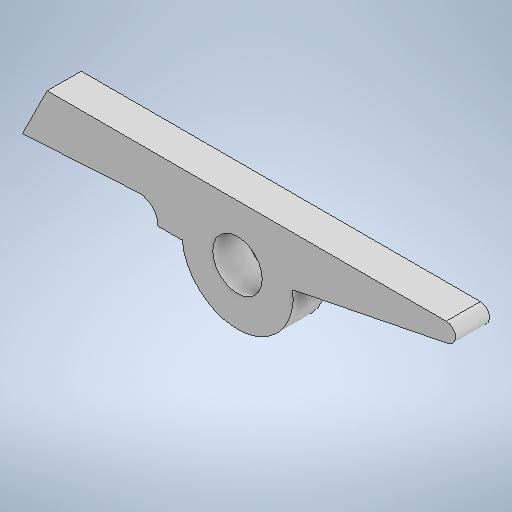
# Autodesk Inventor part: Pieza 4
Saved by Autodesk Inventor 2025.3 (Build 293356030, 356C)
## iProperties
Created: 2025-08-24
Part Number: Pieza 4
Material: Generic
Document SubType Name: Modeling
Designer: PC
Density: 1 g/cm^3
Appearance: Default
Author: PC
Autodesk Inventor part; units mm, degrees
ref_plane "YZ Plane" through (0, 0, 0) normal (1, 0, 0) x (0, 1, 0)
ref_plane "XZ Plane" through (0, 0, 0) normal (0, 1, 0) x (-1, 0, 0)
ref_plane "XY Plane" through (0, 0, 0) normal (0, 0, 1) x (1, 0, 0)
sketch "Sketch1" plane through (0, 0, 0) normal (0, 0, 1) x (1, 0, 0)
  arc A0 (-8.9443, -1) -> (8.9443, 1) centre (0, 0) ccw
  circle A1 centre (0, 0) radius 4
  line L0 (-30.7602, 9) -> (33.7398, 9)
  arc A2 (34.0346, 6.0293) -> (33.7398, 9) centre (33.7398, 7.5) ccw
  line L1 (5.2033, 1) -> (11.259, 1) construction
  line L2 (8.9443, 1) -> (34.0346, 6.0293)
  line L3 (-8.9443, -1) -> (-12.8471, -1)
  line L4 (-30.7602, 9) -> (-34.7602, 1)
  arc A3 (-12.8471, -1) -> (-16.024, 2.1246) centre (-15.8443, -0.87) ccw
  line L5 (-34.7602, 1) -> (-16.024, 2.1246)
  dimension "d0" = 18
  dimension "d1" = 8
  dimension "d2" = 64.5
  dimension "d3" = 3
  dimension "d4" = 9
  dimension "d5" = 8
  dimension "d8" = 10
  dimension "d10" = 4
  dimension "d11" = 8
  constraints: 12 end point, 6 point on circle, 4 centre point, 3 horizontal, 3 tangent, 2 coincident, 1 point on line
  measures "d0" diameter of A0
  measures "d1" diameter of A1
  measures "d2" distance of L0.start L0.end
  measures "d3" diameter of A2
  measures "d4" distance from line of L0 point (0, 0)
  measures "d5" distance between parallel lines of L0 L1
  measures "d8" distance between parallel lines of L3 L0
  measures "d10" horizontal distance of L0.start L4.end
  measures "d11" vertical distance of L0.start L4.end
extrude "Extrusion1" add sketch "Sketch1" along normal blind 5.5
body "Solid1"
